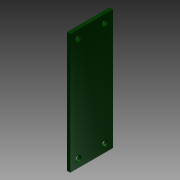
# Autodesk Inventor part: PCBModuleLeft02
Saved by Autodesk Inventor 2013 (Build 170138000, 138)
## iProperties
Created: 2014-07-14
Part Number: PCBModuleLeft02
Material: PCB(1)
Document SubType Name: Modeling
Designer: spichelh
Density: 1 g/cm^3
Author: spichelh
Autodesk Inventor part; units mm, degrees
ref_plane "YZ Plane" through (0, 0, 0) normal (1, 0, 0) x (0, 1, 0)
ref_plane "XZ Plane" through (0, 0, 0) normal (0, 1, 0) x (-1, 0, 0)
ref_plane "XY Plane" through (0, 0, 0) normal (0, 0, 1) x (1, 0, 0)
sketch "Sketch1" plane through (0, 0, 0) normal (1, 0, 0) x (0, 1, 0)
  line L0 (0, 0) -> (57.15, 0)
  line L1 (57.15, 0) -> (57.15, 20.32)
  line L2 (0, 0) -> (0, 20.32)
  line L3 (28.575, 0) -> (28.575, 8.5438) construction
  circle A0 centre (3.81, 3.81) radius 1.4
  circle A1 centre (53.34, 3.81) radius 1.4
  circle A2 centre (53.34, 16.51) radius 1.4
  circle A3 centre (3.81, 16.51) radius 1.4
  line L4 (0, 20.32) -> (57.15, 20.32)
  dimension "d0" = 57.15
  dimension "d1" = 20.32
  dimension "d2" = 20.32
  dimension "d5" = 2.8
  dimension "d6" = 3.81
  dimension "d7" = 3.81
  dimension "d14" = 2.8
  dimension "d15" = 12.7
  dimension "d18" = 49.53
  constraints: 10 end point, 4 centre point, 2 parallel, 2 symmetric about line, 1 horizontal, 1 midpoint, 1 perpendicular, 1 vertical alignment, 2 other
  measures "d0" distance of L0.start L0.end
  measures "d1" distance of L0.end L1.end
  measures "d2" distance of L0.start L2.end
  measures "d5" diameter of A0
  measures "d6" distance from line of L0 A0.centre
  measures "d7" distance from line of L2 A0.centre
  measures "d14" diameter of A2
  measures "d15" distance of A1.centre A2.centre
  measures "d18" distance of A3.centre A2.centre
extrude "Extrusion1" add sketch "Sketch1" along normal blind 1.6
body "Solid1"
